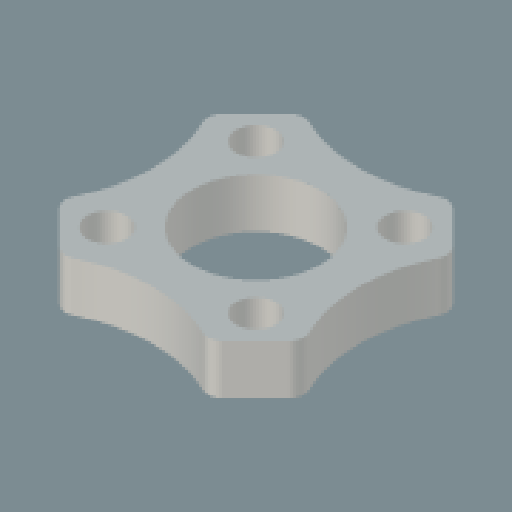
# Autodesk Inventor part: WobbleX WS12
Saved by Autodesk Inventor 2023.2 (Build 272271000, 271)
## iProperties
Created: 2023-02-17
Part Number: WobbleX WS12
Material: Aluminum 6061
Document SubType Name: Modeling
Designer: remop
Density: 2.7 g/cm^3
Appearance: Aluminum - Flat
Author: remop
Autodesk Inventor part; units mm, degrees
ref_plane "YZ Plane" through (0, 0, 0) normal (1, 0, 0) x (0, 1, 0)
ref_plane "XZ Plane" through (0, 0, 0) normal (0, 1, 0) x (-1, 0, 0)
ref_plane "XY Plane" through (0, 0, 0) normal (0, 0, 1) x (1, 0, 0)
sketch "Sketch1" plane through (0, 0, 0) normal (0, 1, 0) x (-1, 0, 0)
  circle A0 centre (0, 0) radius 13
  line L0 (-14.9666, 24.75) -> (-24.75, 14.9666)
  line L1 (-24.75, 14.9666) -> (-24.75, -14.9666) construction
  line L2 (-24.75, -14.9666) -> (-14.9666, -24.75)
  line L3 (-14.9666, -24.75) -> (14.9666, -24.75) construction
  line L4 (14.9666, -24.75) -> (24.75, -14.9666)
  line L5 (24.75, -14.9666) -> (24.75, 14.9666) construction
  line L6 (24.75, 14.9666) -> (14.9666, 24.75)
  line L7 (14.9666, 24.75) -> (-14.9666, 24.75) construction
  arc A1 (-24.75, -14.9666) -> (-24.75, 14.9666) centre (-50.75, 0) ccw
  arc A2 (-14.9666, 24.75) -> (14.9666, 24.75) centre (0, 50.75) ccw
  arc A3 (24.75, 14.9666) -> (24.75, -14.9666) centre (50.75, 0) ccw
  arc A4 (14.9666, -24.75) -> (-14.9666, -24.75) centre (0, -50.75) ccw
  circle A5 centre (-15, 15) radius 4
  circle A6 centre (15, 15) radius 4
  circle A7 centre (15, -15) radius 4
  circle A8 centre (-15, -15) radius 4
  point P0 (-24.75, 0)
  point P1 (24.75, 0)
  point P2 (0, 24.75)
  point P3 (0, -24.75)
  point P4 (0, 20.75)
  dimension "d0" = 26
  dimension "d1" = 49.5
  dimension "d2" = 30
  dimension "d3" = 4
  dimension "d4" = 30
  dimension "d5" = 30
  dimension "d6" = 15
  dimension "d7" = 15
  dimension "d8" = 8
  constraints: 16 end point, 9 centre point, 9 point on circle, 6 equal radius, 6 perpendicular, 4 horizontal alignment, 4 midpoint, 4 vertical alignment, 2 parallel, 2 vertical, 1 coincident, 1 horizontal
  measures "d0" diameter of A0
  measures "d1" distance between parallel lines of L3 L7
  measures "d2" radius of A2
  measures "d3" distance of point (0, 20.75) point (0, 24.75)
  measures "d4" distance of A7.centre A6.centre
  measures "d5" distance of A5.centre A6.centre
  measures "d6" horizontal distance of point (0, 0) A6.centre
  measures "d7" horizontal distance of point (0, 0) A6.centre
  measures "d8" diameter of A6
extrude "Extrusion1" add sketch "Sketch1" along normal blind 7
fillet "Fillet1" radius 3 8 edges at (24.75, 3.5, 14.9666) (14.9666, 3.5, 24.75) (-14.9666, 3.5, 24.75) (-24.75, 3.5, 14.9666) (-24.75, 3.5, -14.9666) (-14.9666, 3.5, -24.75) (14.9666, 3.5, -24.75) (24.75, 3.5, -14.9666)
equation "\"d5\" = d4"
equation "\"d6\" = 0.5 * d5"
equation "\"d7\" = d6"
body "Solid1"
